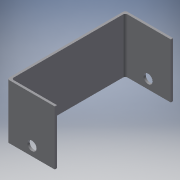
# Autodesk Inventor part: C chanel Short
Saved by Autodesk Inventor 2017 (Build 210142000, 142)
## iProperties
Created: 2019-02-06
Part Number: C chanel Short
Material: Generic
Document SubType Name: Modeling
Designer: S346795925
Density: 1 g/cm^3
Appearance: Default
Author: S346795925
Autodesk Inventor part; units mm, degrees
ref_plane "YZ Plane" through (0, 0, 0) normal (1, 0, 0) x (0, 1, 0)
ref_plane "XZ Plane" through (0, 0, 0) normal (0, 1, 0) x (-1, 0, 0)
ref_plane "XY Plane" through (0, 0, 0) normal (0, 0, 1) x (1, 0, 0)
sketch "Sketch1" plane through (0, 0, 0) normal (0, 1, 0) x (-1, 0, 0)
  line L0 (0, -3.175) -> (0, -155.575)
  line L1 (-3.175, -158.75) -> (-63.5, -158.75)
  line L2 (-3.175, 0) -> (-63.5, 0)
  line L3 (-63.5, -161.925) -> (0, -161.925)
  line L4 (3.175, -158.75) -> (3.175, 0)
  line L5 (0, 3.175) -> (-63.5, 3.175)
  line L6 (-63.5, 0) -> (-63.5, 3.175)
  line L7 (-63.5, -161.925) -> (-63.5, -158.75)
  arc A0 (3.175, 0) -> (0, 3.175) centre (0, 0) ccw
  arc A1 (0, -3.175) -> (-3.175, 0) centre (-3.175, -3.175) ccw
  arc A2 (-3.175, -158.75) -> (0, -155.575) centre (-3.175, -155.575) ccw
  arc A3 (0, -161.925) -> (3.175, -158.75) centre (0, -158.75) ccw
  point P0 (0, 0)
  point P1 (0, -158.75)
  dimension "d0" = 158.75
  dimension "d1" = 63.5
  dimension "d2" = 63.5
  dimension "d3" = 3.175
  dimension "d4" = 3.175
  constraints: 16 end point, 8 point on circle, 8 tangent, 4 centre point, 4 point on line, 3 equal radius, 3 vertical, 2 perpendicular, 1 horizontal, 2 other
  measures "d0" distance of point (0, 0) point (0, -158.75)
  measures "d1" distance of point (0, -158.75) L1.end
  measures "d2" distance of point (0, 0) L2.end
  measures "d3" distance between parallel lines of L0 L4
  measures "d4" radius of A0
extrude "Extrusion1" add sketch "Sketch1" along normal blind 76.2
sketch "Sketch2" plane through (0, 0, 3.175) normal (0, 0, 1) x (1, 0, 0)
  circle A0 centre (31.75, 12.7) radius 6.35
  line L0 (63.5, 0) -> (63.5, 76.2) projected
  line L1 (0, 76.2) -> (63.5, 76.2) projected
  point P0 (0, 0)
  dimension "d7" = 12.7
  dimension "d8" = 31.75
  dimension "d9" = 63.5
  constraints: 1 centre point
  measures "d7" diameter of A0
  measures "d8" distance from line of L0 A0.centre
  measures "d9" distance from line of L1 A0.centre
extrude "Extrusion2" cut sketch "Sketch2" against normal through all
body "Solid1"
